nuxal_reprap4040_Zadjust (Autodesk Fusion 360 design; units mm, degrees)
Autodesk Fusion 360 part; units mm, degrees
sketch "Sketch1" plane through (0, 0, 0) normal (0, 1, 0) x (1, 0, 0)
  line L0 (0, 0) -> (10, 0)
  line L1 (10, 0) -> (10, -20)
  line L2 (10, -20) -> (0, -20)
  line L3 (0, -20) -> (0, 0)
  line L4 (0, -20) -> (10, -20)
  line L5 (10, -20) -> (10, -30)
  line L6 (10, -30) -> (0, -30)
  line L7 (0, -30) -> (0, -20)
  circle A0 centre (5, -5) radius 1.65
  line L8 (8, -23.5) -> (2, -23.5)
  line L9 (2, -23.5) -> (2, -26.5)
  line L10 (2, -26.5) -> (8, -26.5)
  line L11 (8, -26.5) -> (8, -23.5)
  line L12 (8, -23.5) -> (2, -26.5) construction
  line L13 (2, -23.5) -> (8, -26.5) construction
  line L14 (0, -30) -> (10, -30)
  line L15 (10, -30) -> (10, -34)
  line L16 (10, -34) -> (0, -34)
  line L17 (0, -34) -> (0, -30)
  dimension "d1" = 3.3
  dimension "d2" = 6
  dimension "d3" = 3
  constraint horizontal L0
  constraint vertical L1
  constraint horizontal L2
  constraint vertical L3
  constraint coincident L0.start L3.end
  constraint horizontal L4
  constraint vertical L5
  constraint horizontal L6
  constraint vertical L7
  constraint perpendicular L8 L9
  constraint parallel L8 L10
  constraint parallel L9 L11
  constraint horizontal L8
  constraint coincident L12 L0.start
  constraint coincident L13 L0.start
  constraint horizontal L14
  constraint vertical L15
  constraint horizontal L16
  constraint vertical L17
  measures "d1" diameter of A0
  measures "d3" distance of L0.start
extrude "Extrude1" add sketch "Sketch1" along normal blind 5 contours L0 L1 L2 L3 L4
extrude "Extrude2" add sketch "Sketch1" along normal blind 15 contours L2 L4 L5 L6 L7 L14
sketch "Sketch2" plane through (0, 0, 20) normal (0, 0, -1) x (-1, 0, 0)
  line L0 (-10, 5) -> (0, 5)
  line L1 (0, 5) -> (0, 15)
  line L2 (0, 15) -> (-10, 15)
  line L3 (-10, 15) -> (-10, 5)
  circle A0 centre (-5, 10) radius 1.5
  dimension "d8" = 3
  measures "d8" diameter of A0
extrude "Extrude3" add sketch "Sketch1" along normal blind 15 contours L6 L14 L15 L16 L17
extrude "Extrude4" cut sketch "Sketch2" against normal blind 20 contours A0
